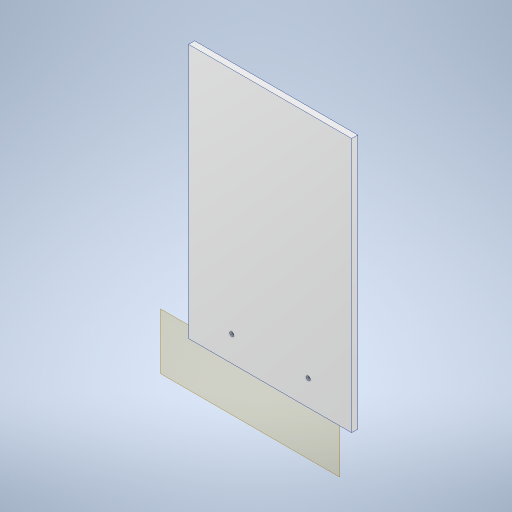
# Autodesk Inventor part: Z axis Back Plate
Saved by Autodesk Inventor 2023.2 (Build 272271000, 271)
## iProperties
Created: 2023-02-15
Part Number: Z axis Back Plate
Material: Aluminum 6061
Document SubType Name: Modeling
Designer: dmargari
Density: 2.7 g/cm^3
Appearance: Aluminum - Flat
Author: dmargari
Autodesk Inventor part; units mm, degrees
ref_plane "YZ Plane" through (0, 0, 0) normal (1, 0, 0) x (0, 1, 0)
ref_plane "XZ Plane" through (0, 0, 0) normal (0, 1, 0) x (-1, 0, 0)
ref_plane "XY Plane" through (0, 0, 0) normal (0, 0, 1) x (1, 0, 0)
ref_plane "Work Plane1" through (0, 0, 0) normal (0, 0, 1) x (1, 0, 0)
sketch "Sketch1" plane through (0, 0, 0) normal (0, 0, 1) x (1, 0, 0)
  line L0 (105.6587, 72.0604) -> (105.6587, 22.0626) projected
  line L1 (-54.3413, 72.0604) -> (105.6587, 72.0604) projected
  line L2 (-54.3413, 22.0626) -> (-54.3413, 72.0604) projected
  line L3 (105.6587, 22.0626) -> (-54.3413, 22.0626) projected
  line L4 (105.6587, 72.0604) -> (105.6587, 272.0604)
  line L5 (105.6587, 272.0604) -> (-54.3413, 272.0604)
  line L6 (-54.3413, 272.0604) -> (-54.3413, 72.0604)
  line L7 (105.6587, 72.0604) -> (-54.3413, 72.0604)
  line L8 (-54.3413, 72.0604) -> (-54.3413, 22.0626)
  line L9 (105.6587, 22.0626) -> (105.6587, 72.0604)
  line L10 (105.6587, 22.0626) -> (-54.3413, 22.0626)
  ellipse E0 centre (-11.8413, 47.0615) end of major axis (-9.7743, 47.0615) minor radius 2.0669 projected
  ellipse E1 centre (63.1587, 47.0615) end of major axis (65.2257, 47.0615) minor radius 2.0669 projected
  ellipse E2 centre (63.1587, 47.0615) end of major axis (65.2257, 47.0615) minor radius 2.0669 projected
  ellipse E3 centre (-11.8413, 47.0615) end of major axis (-9.7743, 47.0615) minor radius 2.0669 projected
  ellipse E4 centre (-36.8413, 63.0608) end of major axis (-30.8413, 63.0608) minor radius 5.9997 projected
  ellipse E5 centre (88.1587, 63.0608) end of major axis (94.1587, 63.0608) minor radius 5.9997 projected
  point P0 (0, 0)
  point P1 (-46.7889, 82.041)
  dimension "d0" = 200
  constraints: 14 end point, 3 collinear, 3 perpendicular, 1 vertical
  measures "d0" distance of L0.start L4.end
extrude "Extrusion1" add sketch "Sketch1" along normal blind 6 contours L0 L3 L2 L1 | L1 L6 L5 L4 | E4 | E5
body "Solid1"
